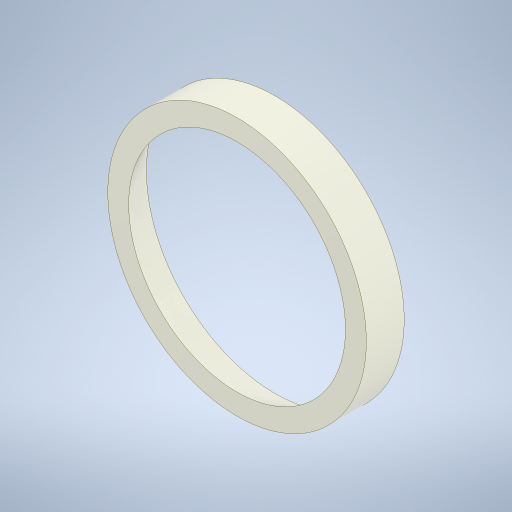
# Autodesk Inventor part: Ring
Saved by Autodesk Inventor 2023.1 (Build 271208000, 208)
## iProperties
Created: 2021-11-02
Part Number: Ring
Material: Polytetrafluoroethylene
Document SubType Name: Modeling
Designer: Timo
Density: 2.02 g/cm^3
Appearance: Smooth - Ivory
Author: Timo
Autodesk Inventor part; units mm, degrees
ref_plane "YZ Plane" through (0, 0, 0) normal (1, 0, 0) x (0, 1, 0)
ref_plane "XZ Plane" through (0, 0, 0) normal (0, 1, 0) x (-1, 0, 0)
ref_plane "XY Plane" through (0, 0, 0) normal (0, 0, 1) x (1, 0, 0)
sketch "Sketch1" plane through (0, 0, 0) normal (1, 0, 0) x (0, 1, 0)
  line L0 (71.65, -0.7523) -> (60.0841, 21)
  line L1 (60.0841, 21) -> (71.65, 21)
  line L2 (71.65, 21) -> (71.65, -0.7523)
  line L3 (-14.33, 0) -> (85.98, 0) projected
  line L4 (0, -5.1027) -> (0, 25.3505) projected
  line L5 (71.65, 0) -> (71.25, 0)
  point P0 (0, 0)
  point P1 (71.65, 0)
  dimension "d0" = 28
  dimension "d2" = 71.65
  dimension "d4" = 0.4
  dimension "d5" = 21
  constraints: 8 end point, 3 point on line, 2 horizontal, 1 perpendicular
  measures "d0" angle of L0 L2
  measures "d2" distance from line of point (0, 0) L2
  measures "d4" distance of L5.start L5.end
  measures "d5" distance between parallel lines of L1 L5
revolve "Revolution1" add sketch "Sketch1" angle 360 about axis through (0, 0, -10) along (0, 0, 1) contours L0 L1 L2 L3
body "Solid1"
